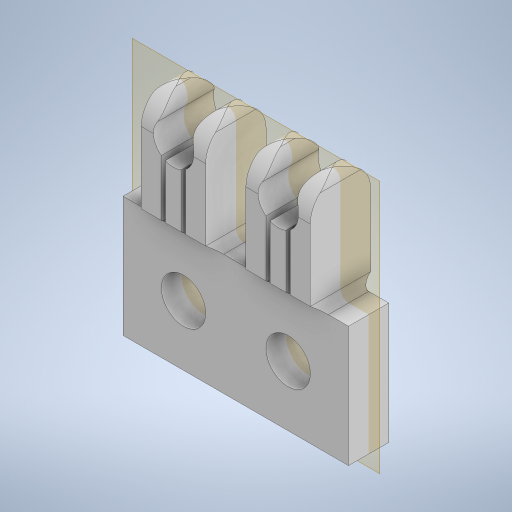
# Autodesk Inventor part: Test fuse holder
Saved by Autodesk Inventor 2024 (Build 280153000, 153)
## iProperties
Created: 2024-04-04
Part Number: Test fuse holder
Material: Generic
Document SubType Name: Modeling
Designer: jens1
Density: 1 g/cm^3
Appearance: Default
Author: jens1
## iProperties of the stored document Test fuse holder_3DPrint.ipt
Created: 2024-04-04
Part Number: Test fuse holder_3DPrint
Material: Generic
Document SubType Name: Modeling
Designer: jens1
Density: 1 g/cm^3
Appearance: Default
Author: jens1
Autodesk Inventor part; units mm, degrees
ref_plane "YZ Plane" through (0, 0, 0) normal (1, 0, 0) x (0, 1, 0)
ref_plane "XZ Plane" through (0, 0, 0) normal (0, 1, 0) x (-1, 0, 0)
ref_plane "XY Plane" through (0, 0, 0) normal (0, 0, 1) x (1, 0, 0)
sketch "Sketch1" plane through (0, 0, 0) normal (0, 0, 1) x (1, 0, 0)
  point P0 (0, 0)
sketch "Sketch2" plane through (0, 0, 0) normal (0, 0, 1) x (1, 0, 0)
  line L0 (0, 0) -> (28, 0)
  line L1 (28, 0) -> (28, 15)
  line L2 (28, 15) -> (0, 15)
  line L3 (0, 15) -> (0, 0)
  line L4 (3.5, 15) -> (3.5, 27.6125)
  line L5 (6, 15) -> (6, 23)
  line L6 (9, 15) -> (9, 23)
  line L7 (11.5, 15) -> (11.5, 27.6125)
  circle A0 centre (7.5, 25) radius 2.25
  circle A1 centre (7.5, 25) radius 2.5
  line L8 (6.5, 15) -> (6.5, 22.7087)
  line L9 (8.5, 15) -> (8.5, 22.7087)
  line L10 (4.9567, 28.5021) -> (7.4, 27.2478)
  line L11 (10.0433, 28.5021) -> (7.6, 27.2478)
  arc A2 (4.9567, 28.5021) -> (3.5, 27.6125) centre (4.5, 27.6125) ccw
  arc A3 (11.5, 27.6125) -> (10.0433, 28.5021) centre (10.5, 27.6125) ccw
  line L12 (0, 0) -> (14, 0)
  line L13 (14, 0) -> (14, 15)
  line L14 (14, 15) -> (0, 15)
  line L15 (0, 15) -> (0, 0)
  line L16 (24.5, 15) -> (24.5, 27.6125)
  line L17 (22, 15) -> (22, 23)
  line L18 (19, 15) -> (19, 23)
  line L19 (16.5, 15) -> (16.5, 27.6125)
  circle A4 centre (20.5, 25) radius 2.25
  circle A5 centre (20.5, 25) radius 2.5
  line L20 (21.5, 15) -> (21.5, 22.7087)
  line L21 (19.5, 15) -> (19.5, 22.7087)
  line L22 (23.0433, 28.5021) -> (20.6, 27.2478)
  line L23 (17.9567, 28.5021) -> (20.4, 27.2478)
  arc A6 (24.5, 27.6125) -> (23.0433, 28.5021) centre (23.5, 27.6125) ccw
  arc A7 (17.9567, 28.5021) -> (16.5, 27.6125) centre (17.5, 27.6125) ccw
  point P0 (3.5, 29.25)
  point P1 (11.5, 29.25)
  point P2 (24.5, 15)
  point P3 (20.9949, 27.4505)
  point P4 (22, 15)
  point P5 (21.5, 15)
  point P6 (19.5, 15)
  point P7 (20.0051, 27.4505)
  point P8 (7.9949, 27.4505)
  point P9 (7.0051, 27.4505)
  dimension "d0" = 28
  dimension "d1" = 15
  dimension "d2" = 4.5
  dimension "d3" = 5
  dimension "d4" = 3.5
  dimension "d5" = 2.5
  dimension "d6" = 2
  dimension "d7" = 1
  dimension "d8" = 2.5
  dimension "d9" = 0.5
  dimension "d10" = 0.5
  dimension "d11" = 0
  dimension "d12" = 0.2
  dimension "d13" = 14.25
  dimension "d14" = 14.25
  dimension "d15" = 10
  dimension "d16" = 1
  dimension "d18" = 15
  dimension "d35" = 13
  constraints: 48 end point, 20 point on circle, 20 symmetric about line, 10 point on line, 8 centre point, 8 parallel, 4 tangent, 2 coincident, 2 horizontal, 2 perpendicular, 2 vertical, 1 equal radius, 4 other
  measures "d0" distance of L2.end L1.end
  measures "d1" distance of L1.end L0.end
  measures "d2" diameter of A0
  measures "d3" diameter of A1
  measures "d4" distance between parallel lines of L4 L3
  measures "d5" distance between parallel lines of L5 L4
  measures "d6" distance between parallel lines of L9 L8
  measures "d7" distance from line of L8 A0.centre
  measures "d8" distance between parallel lines of L7 L6
  measures "d9" distance between parallel lines of L9 L6
  measures "d10" distance between parallel lines of L8 L5
  measures "d11" vertical distance of L10.end L11.end
  measures "d12" distance of L10.end L11.end
  measures "d13" distance of L4.start point (3.5, 29.25)
  measures "d14" distance of L7.start point (11.5, 29.25)
  measures "d15" distance from line of L2 A1.centre
  measures "d16" radius of A2
  measures "d18" distance of L13.end L12.end
  measures "d35" distance of A4.centre A0.centre
extrude "Extrusion1" add sketch "Sketch2" along normal blind 5 contours L3 L2 L13 L0 | L13 L2 L1 L0 | L4 A2 L10 A1 L5 L2 | L19 A7 L23 A5 L18 L2 | L2 L6 A1 L11 A3 L7 | L2 L17 A5 L22 A6 L16 | L8 A1 L9 L2 | L21 A5 L20 L2
fillet "Fillet1" radius 2 4 edges at (7.0051, 27.4505, 2.5) (20.0051, 27.4505, 2.5) (7.9949, 27.4505, 2.5) (20.9949, 27.4505, 2.5)
fillet "Fillet2" radius 1 8 edges at (3.5, 15, 2.5) (6, 15, 2.5) (9, 15, 2.5) (11.5, 15, 2.5) (16.5, 15, 2.5) (19, 15, 2.5) (22, 15, 2.5) (24.5, 15, 2.5)
sketch "Sketch3" plane through (0, 0, 5) normal (0, 0, 1) x (1, 0, 0)
  line L0 (2.5, 15) -> (0, 15) projected
  line L1 (0, 0) -> (28, 0) projected
  line L2 (0, 15) -> (28, 15)
  line L3 (28, 15) -> (28, 0)
  line L4 (28, 0) -> (0, 0)
  line L5 (0, 0) -> (0, 15)
  arc A0 (6.5, 22.7087) -> (8.5, 22.7087) centre (7.5, 25) ccw projected
  arc A1 (19.5, 22.7087) -> (21.5, 22.7087) centre (20.5, 25) ccw projected
  point P0 (7.5, 7.5)
  point P1 (20.5, 7.5)
  dimension "d23" = 0
  dimension "d24" = 0
  dimension "d25" = 0
  dimension "d26" = 15
  dimension "d27" = 7.5
  constraints: 8 end point, 2 parallel, 1 horizontal, 1 perpendicular
  measures "d23" vertical distance of point (20.5, 7.5) point (7.5, 7.5)
  measures "d24" horizontal distance of A0.centre point (7.5, 7.5)
  measures "d25" horizontal distance of A1.centre point (20.5, 7.5)
  measures "d26" distance of L2.end L1.end
  measures "d27" distance from line of L2 point (20.5, 7.5)
hole "Hole1" at (7.5, 7.5, 5) at (20.5, 7.5, 5) direction (0, 0, -1) diameter 5.5 end through all
ref_plane "Work Plane1" through (0, 0, 2.5) normal (0, 0, 1) x (1, 0, 0)
sketch "Sketch4" plane through (0, 0, 2.5) normal (0, 0, 1) x (1, 0, 0)
  circle A0 centre (20.5, 7.5) radius 2.75 projected
  circle A1 centre (7.5, 7.5) radius 2.75 projected
  arc A2 (23.0433, 28.5021) -> (22.709, 26.1705) centre (24.4763, 27.107) ccw projected
  arc A3 (22, 23) -> (22.709, 26.1705) centre (20.5, 25) ccw projected
  line L0 (22, 23) -> (22, 15.866) projected
  arc A4 (21.5, 15) -> (22, 15.866) centre (21, 15.866) ccw projected
  line L1 (21.5, 15) -> (21.5, 22.7087) projected
  arc A5 (19.5, 22.7087) -> (21.5, 22.7087) centre (20.5, 25) ccw projected
  line L2 (19.5, 22.7087) -> (19.5, 15) projected
  arc A6 (19, 15.866) -> (19.5, 15) centre (20, 15.866) ccw projected
  line L3 (19, 15.866) -> (19, 23) projected
  arc A7 (18.291, 26.1705) -> (19, 23) centre (20.5, 25) ccw projected
  arc A8 (18.291, 26.1705) -> (17.9567, 28.5021) centre (16.5237, 27.107) ccw projected
  arc A9 (17.9567, 28.5021) -> (16.5, 27.6125) centre (17.5, 27.6125) ccw projected
  line L4 (16.5, 27.6125) -> (16.5, 16) projected
  arc A10 (15.5, 15) -> (16.5, 16) centre (15.5, 16) ccw projected
  line L5 (15.5, 15) -> (12.5, 15) projected
  arc A11 (11.5, 16) -> (12.5, 15) centre (12.5, 16) ccw projected
  line L6 (11.5, 16) -> (11.5, 27.6125) projected
  arc A12 (11.5, 27.6125) -> (10.0433, 28.5021) centre (10.5, 27.6125) ccw projected
  arc A13 (10.0433, 28.5021) -> (9.709, 26.1705) centre (11.4763, 27.107) ccw projected
  arc A14 (9, 23) -> (9.709, 26.1705) centre (7.5, 25) ccw projected
  line L7 (9, 23) -> (9, 15.866) projected
  arc A15 (8.5, 15) -> (9, 15.866) centre (8, 15.866) ccw projected
  line L8 (8.5, 15) -> (8.5, 22.7087) projected
  arc A16 (6.5, 22.7087) -> (8.5, 22.7087) centre (7.5, 25) ccw projected
  line L9 (6.5, 22.7087) -> (6.5, 15) projected
  arc A17 (6, 15.866) -> (6.5, 15) centre (7, 15.866) ccw projected
  line L10 (6, 15.866) -> (6, 23) projected
  arc A18 (5.291, 26.1705) -> (6, 23) centre (7.5, 25) ccw projected
  arc A19 (5.291, 26.1705) -> (4.9567, 28.5021) centre (3.5237, 27.107) ccw projected
  arc A20 (4.9567, 28.5021) -> (3.5, 27.6125) centre (4.5, 27.6125) ccw projected
  line L11 (3.5, 27.6125) -> (3.5, 16) projected
  arc A21 (2.5, 15) -> (3.5, 16) centre (2.5, 16) ccw projected
  line L12 (2.5, 15) -> (0, 15) projected
  line L13 (0, 15) -> (0, 0) projected
  line L14 (0, 0) -> (28, 0) projected
  line L15 (28, 0) -> (28, 15) projected
  line L16 (28, 15) -> (25.5, 15) projected
  arc A22 (24.5, 16) -> (25.5, 15) centre (25.5, 16) ccw projected
  line L17 (24.5, 16) -> (24.5, 27.6125) projected
  arc A23 (24.5, 27.6125) -> (23.0433, 28.5021) centre (23.5, 27.6125) ccw projected
  line L18 (0, 15) -> (28, 15)
  constraints: 2 end point, 1 horizontal
extrude "Extrusion2" add sketch "Sketch4" along normal mid plane 7.5 contours A23 L17 A22 L18 A4 L0 A3 A2 | L18 L2 A5 L1 | L18 A10 L4 A9 A8 A7 L3 A6 | L18 A15 L7 A14 A13 A12 L6 A11 | L18 L9 A16 L8 | A21 L11 A20 A19 A18 L10 A17 L18
sketch "Sketch5" plane through (3.5, 16, 6.25) normal (-1, 0, 0) x (0, 0, 1)
  line L0 (-6.25, -1) -> (-1.25, -1) projected
  line L1 (-1.25, -1) -> (0, -1) projected
  line L2 (0, 0) -> (0, -1) projected
  line L3 (0, 0) -> (-7.5, 0) projected
  line L4 (-7.5, -1) -> (-7.5, 0) projected
  line L5 (-7.5, -1) -> (-6.25, -1) projected
  line L6 (0, 0) -> (-7.5, 0) projected
  line L7 (0, 11.6125) -> (0, 0) projected
  line L8 (-7.5, 11.6125) -> (0, 11.6125) projected
  line L9 (-7.5, 0) -> (-7.5, 11.6125) projected
  line L10 (-6.25, -1) -> (-6.25, -16) projected
  line L11 (-6.25, -16) -> (-1.25, -16) projected
  line L12 (-1.25, -1) -> (-1.25, -16) projected
  line L13 (-6.25, -1) -> (-1.25, -1) projected
  line L14 (-7.5, 0) -> (-6.25, -1)
  line L15 (-1.25, -1) -> (0, 0)
  constraints: 4 end point
extrude "Extrusion3" cut sketch "Sketch5" along normal blind 100 and the other way blind 100 contours L5 L4 L14 | L15 L2 L1
sketch "Sketch6" plane through (3.5, 27.6125, -1.25) normal (-1, 0, 0) x (0, 0, 1)
  line L0 (0, 1) -> (7.5, 1) projected
  line L1 (7.5, -4.6125) -> (7.5, -11.6125) projected
  line L2 (0, 1) -> (7.5, 1)
  line L3 (7.5, 1) -> (7.5, -11.6125)
  line L4 (7.5, -11.6125) -> (0, -11.6125)
  line L5 (0, -11.6125) -> (0, 1)
  circle A0 centre (3.75, -2.75) radius 3.75
  circle A1 centre (3.75, -2.75) radius 3.75
  line L6 (0, -11.6125) -> (0, 0) projected
  line L7 (7.5, 0) -> (7.5, -11.6125) projected
  line L8 (3.3964, 0.6464) -> (0, -2.75)
  line L9 (4.1036, 0.6464) -> (7.5, -2.75)
  arc A2 (4.1036, 0.6464) -> (3.3964, 0.6464) centre (3.75, 0.2929) ccw
  point P0 (1.25, -27.6125)
  point P1 (3.75, 1)
  point P2 (3.75, 1)
  point P3 (3.75, 1)
  point P4 (7.5, -2.75)
  point P5 (0, -2.75)
  dimension "d45" = 7.5
  dimension "d43" = 0
  dimension "d44" = 7.5
  dimension "d48" = 0.5
  constraints: 12 end point, 5 point on circle, 4 point on line, 4 tangent, 2 centre point, 2 horizontal, 2 midpoint, 2 parallel, 1 perpendicular, 1 vertical, 3 other
  measures "d43" distance of point (3.75, -2.75) A1.centre
  measures "d44" distance of L0.start L0.end
  measures "d48" radius of A2
extrude "Extrusion4" cut sketch "Sketch6" against normal through all contours L0 A0 L5 | L0 L3 A0
equation "\"d9\" = d10"
equation "\"d14\" = d13"
equation "\"d18\" = d1"
equation "\"d27\" = 0.5 * d26"
equation "\"d45\" = d44"
body "Solid1"
